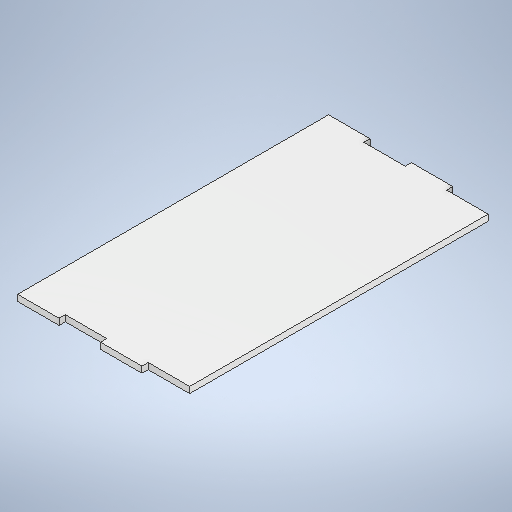
# Autodesk Inventor part: base prt 2 N
Saved by Autodesk Inventor 2025.3 (Build 293356000, 356)
## iProperties
Created: 2026-04-06
Part Number: base prt 2 N
Material: ABS Plastic
Document SubType Name: Modeling
Designer: logien
Density: 1.06 g/cm^3
Appearance: Smooth - White
Author: logien
Autodesk Inventor part; units mm, degrees
ref_plane "YZ Plane" through (0, 0, 0) normal (1, 0, 0) x (0, 1, 0)
ref_plane "XZ Plane" through (0, 0, 0) normal (0, 1, 0) x (-1, 0, 0)
ref_plane "XY Plane" through (0, 0, 0) normal (0, 0, 1) x (1, 0, 0)
sketch "Sketch1" plane through (0, 0, 0) normal (0, 1, 0) x (-1, 0, 0)
  line L0 (0, 0) -> (0, -144)
  line L1 (0, 0) -> (20, 0)
  line L2 (20, 0) -> (20, 3)
  line L3 (20, 3) -> (40, 3)
  line L4 (40, 3) -> (40, 0)
  line L5 (40, 0) -> (60, 0)
  line L6 (60, 0) -> (60, 3)
  line L7 (60, 3) -> (80, 3)
  line L8 (0, -72) -> (20, -72)
  line L9 (0, -144) -> (20, -144)
  line L10 (20, -144) -> (20, -147)
  line L11 (20, -147) -> (40, -147)
  line L12 (40, -147) -> (40, -144)
  line L13 (40, -144) -> (60, -144)
  line L14 (60, -144) -> (60, -147)
  line L15 (60, -147) -> (80, -147)
  line L16 (80, 3) -> (80, -147)
  dimension "d0" = 144
  dimension "d1" = 20
  dimension "d2" = 3
  dimension "d3" = 20
  dimension "d4" = 20
  dimension "d5" = 20
  dimension "d6" = 20
  constraints: 34 end point, 7 symmetric about line, 6 point on line, 4 perpendicular, 3 horizontal, 2 vertical, 1 midpoint
  measures "d0" distance of L0.start L0.end
  measures "d1" distance of L0.start L1.end
  measures "d2" distance of L1.end L2.end
  measures "d3" distance of L2.end L3.end
  measures "d4" distance of L4.end L5.end
  measures "d5" distance of L6.end L7.end
  measures "d6" distance of L8.start L8.end
extrude "Extrusion1" add sketch "Sketch1" along normal blind 3
body "Solid1"
